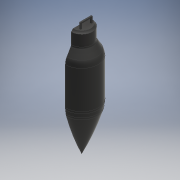
# Autodesk Inventor part: noze-cone-side-2
Saved by Autodesk Inventor 2017 (Build 210142000, 142)
## iProperties
Created: 2020-06-18
Part Number: noze-cone-side-2
Material: Polycarbonate, Clear
Document SubType Name: Modeling
Designer: HAYNIE R&D
Density: 1.2 g/cm^3
Appearance: Smooth - Black
Mass: 17.4989 g
Surface Area: 267.995 cm^2
Volume: 14.5824 cm^3
Author: HAYNIE R&D
Autodesk Inventor part; units mm, degrees
ref_plane "YZ Plane" through (0, 0, 0) normal (1, 0, 0) x (0, 1, 0)
ref_plane "XZ Plane" through (0, 0, 0) normal (0, 1, 0) x (-1, 0, 0)
ref_plane "XY Plane" through (0, 0, 0) normal (0, 0, 1) x (1, 0, 0)
sketch "Sketch1" plane through (0, 0, 0) normal (1, 0, 0) x (0, 1, 0)
  line L0 (0, 0) -> (0, -200)
  line L1 (17.75, -33.271) -> (27.75, -50.5915)
  line L2 (27.75, -50.5915) -> (27.75, -125.5915)
  line L3 (16.75, -33.271) -> (26.75, -50.5915)
  line L4 (16.75, -33.271) -> (36.75, -33.271) construction
  line L5 (26.75, -50.5915) -> (26.75, -125.5915)
  line L6 (17.75, -33.271) -> (17.75, -13.271)
  line L7 (16.75, -13.271) -> (32.074, -13.271) construction
  line L8 (17.75, -13.271) -> (33.074, -13.271) construction
  line L9 (17.75, -13.271) -> (33.074, -13.271) construction
  line L10 (16.75, -13.271) -> (31.4966, -13.271) construction
  line L11 (16.75, -33.271) -> (16.75, -14.271)
  line L12 (16.75, -14.271) -> (0, -14.271)
  line L13 (17.75, -13.271) -> (0, -13.271)
  arc A0 (0, -200) -> (27.75, -125.5915) centre (-356.6732, -24.6031) ccw
  line L14 (0, -200) -> (0, -199)
  arc A1 (0, -199) -> (26.75, -125.5915) centre (-482.9464, 18.5633) ccw
  line L15 (0, -200) -> (0, -199)
  point P0 (0, -1)
  dimension "d0" = 200
  dimension "d7" = 75
  dimension "d31" = 19
  constraints: 32 end point, 5 horizontal, 5 point on line, 5 vertical, 4 point on circle, 2 centre point, 1 collinear, 1 equal length, 1 perpendicular
  measures "d0" distance of L0.start L0.end
  measures "d7" distance of L1.end L2.end
  measures "d31" distance of L3.start L11.end
revolve "Revolution2" add sketch "Sketch1" angle 360 about axis through (0, 0, 0) along (0, 0, -1) contours L13 L6 L1 L2 A0 L0 A1 L5 L3 L11 L12
fillet "Fillet5" radius 5 1 edges at (0, -17.75, -33.271)
sketch "Sketch4" plane through (0, 0, -13.271) normal (0, 0, 1) x (1, 0, 0)
  circle A0 centre (0, 0) radius 15
  dimension "d36" = 30
  constraints: 1 centre point, 1 coincident
  measures "d36" diameter of A0
extrude "Extrusion2" add sketch "Sketch4" along normal blind 3.27
split "Split3" plane through (0, 0, 0) removes the side toward (-1, 0, 0)
fillet "Fillet8" radius 20 1 edges at (27.75, 0, -50.5915)
fillet "Fillet10" radius 10 1 edges at (15, 0, -13.271)
sketch "Sketch8" plane through (0, 0, -10.001) normal (0, 0, 1) x (1, 0, 0)
  line L0 (8, -10) -> (6, -10)
  line L1 (6, -10) -> (6, -8)
  line L2 (6, -8) -> (8, -8)
  line L3 (8, -8) -> (8, -10)
  line L4 (8, 8) -> (6, 8)
  line L5 (6, 8) -> (6, 10)
  line L6 (6, 10) -> (8, 10)
  line L7 (8, 10) -> (8, 8)
  point P0 (0, 0)
  dimension "d49" = 16
  constraints: 16 end point, 4 parallel, 2 horizontal, 2 perpendicular
  measures "d49" distance of L4.end L1.end
extrude "Extrusion5" add sketch "Sketch8" along normal blind 10
sketch "Sketch9" plane through (0, 0, -0.001) normal (0, 0, 1) x (1, 0, 0)
  line L0 (6, 10) -> (8, 10) projected
  line L1 (8, -10) -> (6, -10)
  line L2 (6, -10) -> (6, 10)
  line L3 (6, 10) -> (8, 10)
  line L4 (8, 10) -> (8, -10)
  point P0 (0, 0)
  constraints: 8 end point, 2 parallel, 1 horizontal, 1 perpendicular
extrude "Extrusion6" add sketch "Sketch9" against normal blind 2
chamfer "Chamfer1" distance 2 angle 45 1 edges at (26.75, 0, -50.5915)
chamfer "Chamfer2" distance 2 angle 45 1 edges at (26.75, 0, -125.5915)
chamfer "Chamfer3" distance 5 angle 45 1 edges at (27.75, 0, -125.5915)
fillet "Fillet15" radius 25 1 edges at (27.75, 0, -120.5915)
fillet "Fillet16" radius 25 1 edges at (26.4492, 0, -130.4192)
